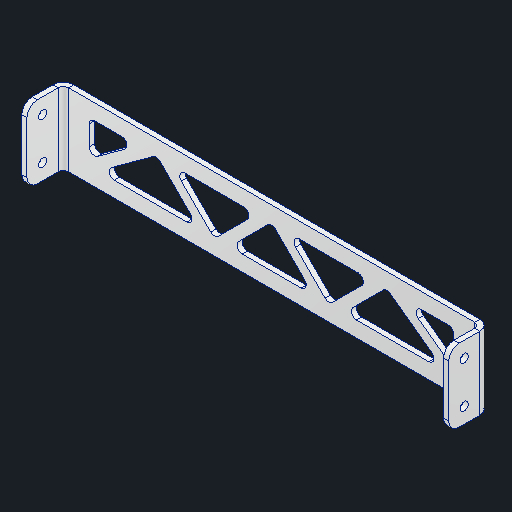
# Autodesk Inventor part: feeder_middle_brace
Saved by Autodesk Inventor 2024.3 (Build 283343010, 343A)
## iProperties
Created: 2025-03-09
Part Number: feeder_middle_brace
Material: Aluminum 6061
Document SubType Name: Sheet Metal
Designer: marcu
Density: 2.7 g/cm^3
Sheet Metal Rule: Default
Appearance: Aluminum - Flat
Mass: 79.3609 g
Surface Area: 231.149 cm^2
Volume: 29.3929 cm^3
Author: marcu
Autodesk Inventor part; units mm, degrees
ref_plane "YZ Plane" through (0, 0, 0) normal (1, 0, 0) x (0, 1, 0)
ref_plane "XZ Plane" through (0, 0, 0) normal (0, 1, 0) x (-1, 0, 0)
ref_plane "XY Plane" through (0, 0, 0) normal (0, 0, 1) x (1, 0, 0)
sketch "Sketch1" plane through (0, 0, 0) normal (0, 0, 1) x (1, 0, 0)
  line L0 (130.429, -22.225) -> (-130.429, -22.225)
  line L1 (-130.429, -22.225) -> (-130.429, 22.225)
  line L2 (-130.429, 22.225) -> (130.429, 22.225)
  line L3 (130.429, 22.225) -> (130.429, -22.225)
  line L4 (130.429, -22.225) -> (-130.429, 22.225) construction
  line L5 (-130.429, -22.225) -> (130.429, 22.225) construction
  point P0 (0, 0)
  dimension "d0" = 260.858
  dimension "d1" = 44.45
  measures "d0" distance of L1.end L2.end
  measures "d1" distance of L0.end L1.end
extrude "Plate1" add sketch "Sketch1" along normal blind 3.175
sketch "Sketch2" plane through (-127.254, -22.225, 0) normal (-1, 0, 0) x (0, -1, 0)
  line L0 (-44.45, 0) -> (0, 0)
  line L1 (0, 0) -> (0, 25.4)
  line L2 (0, 25.4) -> (-44.45, 25.4)
  line L3 (-44.45, 25.4) -> (-44.45, 0)
  constraints: 6 end point, 1 horizontal, 1 perpendicular, 1 vertical
edge flange "Flange1" height 25.4 angle 90 thickness 3.175 bend radius 3.175 thickness toward (-1, 0, 0) relief straight relief width 3.175 relief depth 1.5875 corner gap 3.175 corner form 0 edges at (-130.429, 0, 3.175) (130.429, 0, 3.175) wall of the first edge with corners at (-127.254, 22.225, 0) (-127.254, -22.225, 0) (-127.254, -22.225, 25.4) (-127.254, 22.225, 25.4)
bend "Bend1"
corner "Corner1"
sketch "Sketch3" plane through (-130.429, -22.225, 25.4) normal (-1, 0, 0) x (0, 0, 1)
  line L0 (0, 44.45) -> (0, 0) construction
  line L1 (-9.525, 9.525) -> (-9.525, 34.925) construction
  point P0 (-25.4, 22.225)
  point P1 (-9.525, 22.225)
  dimension "d13" = 25.4
  dimension "d14" = 9.525
  constraints: 2 end point, 1 horizontal alignment, 1 midpoint, 1 vertical, 1 vertical alignment
  measures "d13" distance of L1.end L1.start
  measures "d14" distance from line of L0 L1.start
hole "Hole1" at (-130.429, -12.7, 15.875) at (-130.429, 12.7, 15.875) direction (1, 0, 0) diameter 5.1054 end through all clearance for "Flat Head Machine Screw (82)" size "#10" standard "Ansi Unified Screw Threads"
sketch "Sketch4" plane through (0, 0, 0) normal (0, 0, -1) x (-1, 0, 0)
  line L0 (-117.729, 15.875) -> (-117.729, -15.875) construction
  line L1 (-124.079, 15.875) -> (-124.079, -15.875)
  line L2 (-111.379, -15.875) -> (-111.379, 15.875)
  arc A0 (-111.379, 15.875) -> (-124.079, 15.875) centre (-117.729, 15.875) ccw
  arc A1 (-124.079, -15.875) -> (-111.379, -15.875) centre (-117.729, -15.875) ccw
  line L3 (-124.079, 22.225) -> (124.079, 22.225) projected
  line L4 (124.079, -22.225) -> (-124.079, -22.225) projected
  line L5 (-124.079, 22.225) -> (-124.079, -22.225) projected
  line L6 (-119.3165, 17.4625) -> (119.3165, 17.4625) construction
  line L7 (-119.3165, 12.7) -> (119.3165, 12.7)
  line L8 (119.3165, 22.225) -> (-119.3165, 22.225)
  arc A2 (-119.3165, 22.225) -> (-119.3165, 12.7) centre (-119.3165, 17.4625) ccw
  arc A3 (119.3165, 12.7) -> (119.3165, 22.225) centre (119.3165, 17.4625) ccw
  line L9 (124.079, -22.225) -> (124.079, 22.225) projected
  line L10 (119.3165, -17.4625) -> (-119.3165, -17.4625) construction
  line L11 (119.3165, -12.7) -> (-119.3165, -12.7)
  line L12 (-119.3165, -22.225) -> (119.3165, -22.225)
  arc A4 (119.3165, -22.225) -> (119.3165, -12.7) centre (119.3165, -17.4625) ccw
  arc A5 (-119.3165, -12.7) -> (-119.3165, -22.225) centre (-119.3165, -17.4625) ccw
  line L13 (117.729, 15.875) -> (117.729, -15.875) construction
  line L14 (111.379, 15.875) -> (111.379, -15.875)
  line L15 (124.079, -15.875) -> (124.079, 15.875)
  arc A6 (124.079, 15.875) -> (111.379, 15.875) centre (117.729, 15.875) ccw
  arc A7 (111.379, -15.875) -> (124.079, -15.875) centre (117.729, -15.875) ccw
  line L16 (0, 17.4625) -> (-34.925, -17.4625) construction
  line L17 (-2.2451, 19.7076) -> (-37.1701, -15.2174)
  line L18 (-32.6799, -19.7076) -> (2.2451, 15.2174)
  arc A8 (2.2451, 15.2174) -> (-2.2451, 19.7076) centre (0, 17.4625) ccw
  arc A9 (-37.1701, -15.2174) -> (-32.6799, -19.7076) centre (-34.925, -17.4625) ccw
  line L19 (0, 17.4625) -> (49.3914, 17.4625) construction
  line L20 (-34.925, -17.4625) -> (-69.85, 17.4625) construction
  line L21 (-32.6799, -15.2174) -> (-67.6049, 19.7076)
  line L22 (-72.0951, 15.2174) -> (-37.1701, -19.7076)
  arc A10 (-37.1701, -19.7076) -> (-32.6799, -15.2174) centre (-34.925, -17.4625) ccw
  arc A11 (-67.6049, 19.7076) -> (-72.0951, 15.2174) centre (-69.85, 17.4625) ccw
  line L23 (-34.925, -17.4625) -> (14.4664, -17.4625) construction
  line L24 (-69.85, 17.4625) -> (-117.729, -17.4625) construction
  line L25 (-71.7211, 20.0276) -> (-119.6001, -14.8974)
  line L26 (-115.8579, -20.0276) -> (-67.9789, 14.8974)
  arc A12 (-67.9789, 14.8974) -> (-71.7211, 20.0276) centre (-69.85, 17.4625) ccw
  arc A13 (-119.6001, -14.8974) -> (-115.8579, -20.0276) centre (-117.729, -17.4625) ccw
  line L27 (0, 17.4625) -> (34.925, -17.4625) construction
  line L28 (-2.2451, 15.2174) -> (32.6799, -19.7076)
  line L29 (37.1701, -15.2174) -> (2.2451, 19.7076)
  arc A14 (2.2451, 19.7076) -> (-2.2451, 15.2174) centre (0, 17.4625) ccw
  arc A15 (32.6799, -19.7076) -> (37.1701, -15.2174) centre (34.925, -17.4625) ccw
  line L30 (0, 17.4625) -> (49.3914, 17.4625) construction
  line L31 (34.925, -17.4625) -> (69.85, 17.4625) construction
  line L32 (37.1701, -19.7076) -> (72.0951, 15.2174)
  line L33 (67.6049, 19.7076) -> (32.6799, -15.2174)
  arc A16 (32.6799, -15.2174) -> (37.1701, -19.7076) centre (34.925, -17.4625) ccw
  arc A17 (72.0951, 15.2174) -> (67.6049, 19.7076) centre (69.85, 17.4625) ccw
  line L34 (34.925, -17.4625) -> (84.3164, -17.4625) construction
  line L35 (69.85, 17.4625) -> (117.729, -17.4625) construction
  line L36 (67.9789, 14.8974) -> (115.8579, -20.0276)
  line L37 (119.6001, -14.8974) -> (71.7211, 20.0276)
  arc A18 (71.7211, 20.0276) -> (67.9789, 14.8974) centre (69.85, 17.4625) ccw
  arc A19 (115.8579, -20.0276) -> (119.6001, -14.8974) centre (117.729, -17.4625) ccw
  point P0 (0, 0)
  point P1 (-117.729, 0)
  point P2 (0, -17.4625)
  point P3 (117.729, 0)
  point P4 (-17.4625, 0)
  point P5 (-52.3875, 0)
  point P6 (-93.7895, 0)
  point P7 (17.4625, 0)
  point P8 (52.3875, 0)
  point P9 (93.7895, 0)
  point P10 (81.7665, 12.7)
  point P11 (111.379, -8.9006)
  point P12 (111.379, 12.7)
  point P13 (105.8125, -12.7)
  point P14 (70.1739, 13.2963)
  point P15 (44.1776, -12.7)
  point P16 (34.925, -12.9724)
  point P17 (60.5974, 12.7)
  point P18 (9.2526, 12.7)
  point P19 (25.6724, -12.7)
  point P20 (0, 12.9724)
  point P21 (-25.6724, -12.7)
  point P22 (-60.5974, 12.7)
  point P23 (-34.925, -12.9724)
  point P24 (-9.2526, 12.7)
  point P25 (-70.1739, 13.2963)
  point P26 (-105.8125, -12.7)
  point P27 (-44.1776, -12.7)
  point P28 (-111.379, -8.9006)
  point P29 (-81.7665, 12.7)
  point P30 (-111.379, 12.7)
  dimension "d22" = 12.7
  dimension "d23" = 9.525
  dimension "d24" = 9.525
  dimension "d25" = 12.7
  dimension "d26" = 135
  dimension "d27" = 6.35
  dimension "d28" = 135
  dimension "d29" = 6.35
  dimension "d30" = 6.35
  dimension "d31" = 45
  dimension "d32" = 6.35
  dimension "d33" = 45
  dimension "d34" = 6.35
  dimension "d35" = 6.35
  constraints: 88 end point, 55 tangent, 40 point on circle, 20 centre point, 10 midpoint, 10 parallel, 8 point on line, 4 equal length, 4 horizontal, 1 vertical
  measures "d22" diameter of A1
  measures "d23" diameter of A3
  measures "d24" diameter of A5
  measures "d25" diameter of A7
  measures "d26" angle of L16 L19
  measures "d27" diameter of A9
  measures "d28" angle of L23 L20
  measures "d29" diameter of A11
  measures "d30" diameter of A13
  measures "d31" angle of L27 L30
  measures "d32" diameter of A15
  measures "d33" angle of L34 L31
  measures "d34" diameter of A17
  measures "d35" diameter of A19
extrude "Extrusion1" cut sketch "Sketch4" against normal through all contours L7 L25 L2 | L26 L7 L22 L11 | L14 L37 L7 | L26 L22 L7 | L11 L32 L7 L36 | L21 L7 L17 L11 | L11 L17 L21 | L7 L32 L36 | L33 L29 L11 | L11 L29 L7 L33 | L18 L7 L28 L11 | L18 L28 L7
fillet "Corner Round1" radius 3.175 21 edges at (111.379, 12.7, 1.5875) (111.379, -8.9006, 1.5875) (81.7665, 12.7, 1.5875) (70.1739, 13.2963, 1.5875) (105.8125, -12.7, 1.5875) (44.1776, -12.7, 1.5875) (34.925, -12.9724, 1.5875) (60.5974, 12.7, 1.5875) (9.2526, 12.7, 1.5875) (0, 12.9724, 1.5875) (-25.6724, -12.7, 1.5875) (25.6724, -12.7, 1.5875) (-9.2526, 12.7, 1.5875) (-34.925, -12.9724, 1.5875) (-60.5974, 12.7, 1.5875) (-70.1739, 13.2963, 1.5875) (-105.8125, -12.7, 1.5875) (-44.1776, -12.7, 1.5875) (-81.7665, 12.7, 1.5875) (-111.379, 12.7, 1.5875) (-111.379, -8.9006, 1.5875)
fillet "Corner Round1" radius 6.35 4 edges at (128.8415, 22.225, 25.4) (128.8415, -22.225, 25.4) (-128.8415, 22.225, 25.4) (-128.8415, -22.225, 25.4)
equation "\"d20\" = Thickness"
equation "\"d2\" = Thickness"
equation "\"d3\" = BendReliefWidth"
equation "\"d4\" = BendReliefDepth"
equation "\"d5\" = MinimumRemnant"
equation "\"d6\" = TransitionRadius"
equation "\"d9\" = BendRadius"
equation "\"d10\" = CornerReliefSize"
equation "\"d11\" = GapSize"
equation "\"d12\" = JacobiRadiusSize"
equation "\"BendRadius\" = Thickness"
equation "\"BendReliefWidth\" = Thickness"
equation "\"BendReliefDepth\" = 0.5 * Thickness"
equation "\"CornerReliefSize\" = 4 * Thickness"
equation "\"MinimumRemnant\" = 2 * Thickness"
equation "\"TransitionRadius\" = BendRadius"
equation "\"JacobiRadiusSize\" = BendRadius"
equation "\"GapSize\" = Thickness"
equation "\"Thickness\" = 3.175"
body "Solid1"
